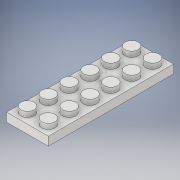
# Autodesk Inventor part: 2x6 short white pegged
Saved by Autodesk Inventor 2017 (Build 210142000, 142)
## iProperties
Created: 2018-05-09
Part Number: 2x6 short white pegged
Material: ABS Plastic
Document SubType Name: Modeling
Designer: Kyle
Density: 1.06 g/cm^3
Appearance: Smooth - White
Author: Kyle
Autodesk Inventor part; units mm, degrees
ref_plane "YZ Plane" through (0, 0, 0) normal (1, 0, 0) x (0, 1, 0)
ref_plane "XZ Plane" through (0, 0, 0) normal (0, 1, 0) x (-1, 0, 0)
ref_plane "XY Plane" through (0, 0, 0) normal (0, 0, 1) x (1, 0, 0)
sketch "Sketch1" plane through (0, 0, 0) normal (0, 1, 0) x (-1, 0, 0)
  line L0 (0, 0) -> (15.5956, 0)
  line L1 (15.5956, 0) -> (15.5956, -46.7868)
  line L2 (15.5956, -46.7868) -> (0, -46.7868)
  line L3 (0, -46.7868) -> (0, 0)
  dimension "d0" = 15.5956
  dimension "d7" = 46.7868
  constraints: 8 end point, 2 parallel, 1 horizontal, 1 perpendicular
  measures "d0" distance of L1.end L2.end
  measures "d7" distance of L0.end L1.end
extrude "Extrusion1" add sketch "Sketch1" along normal blind 3.236
sketch "Sketch2" plane through (0, 3.236, 0) normal (0, 1, 0) x (1, 0, 0)
  line L0 (-15.5956, 0) -> (0, 0) construction
  line L1 (-15.5956, 0) -> (-11.6967, 0) construction
  line L2 (-11.6967, 0) -> (-11.6967, 3.8989) construction
  line L3 (-11.6967, 3.8989) -> (-15.5956, 3.8989) construction
  line L4 (-15.5956, 3.8989) -> (-15.5956, 0) construction
  circle A0 centre (-11.6967, 3.8989) radius 2.4498
  dimension "d10" = 3.8989
  dimension "d11" = 3.8989
  dimension "d12" = 4.8997
  constraints: 8 end point, 2 parallel, 1 centre point, 1 coincident, 1 horizontal, 1 perpendicular
  measures "d10" distance of L3.end L2.end
  measures "d11" distance of L2.end L1.end
  measures "d12" diameter of A0
extrude "Extrusion2" add sketch "Sketch2" along normal blind 1.9837
pattern_linear "Rectangular Pattern1" count 6 spacing 7.7978 along (0, 0, -1) count 2 spacing 7.7978 along (1, 0, 0) of "Extrusion2"
shell "Shell1" thickness 1.4732 removed faces 1 at (-5.1985, 0, -31.1912)
sketch "Sketch3" plane through (-14.1224, 1.7628, -1.4732) normal (0, -1, 0) x (1, 0, 0)
  circle A0 centre (10.2235, -2.4257) radius 2.4498 construction
  circle A1 centre (2.4257, -10.2235) radius 2.4498 construction
  line L0 (10.2235, -2.4257) -> (2.4257, -10.2235) construction
  circle A2 centre (6.3246, -6.3246) radius 3.064
  circle A3 centre (6.3246, -6.3246) radius 2.4498
  point P0 (14.1224, 1.4732)
  dimension "d22" = 4.8997
  constraints: 2 centre point, 2 end point, 1 coincident, 1 midpoint
  measures "d22" diameter of A3
extrude "Extrusion3" add sketch "Sketch3" along normal up to surface (1.7628 mm away)
pattern_linear "Rectangular Pattern2" count 5 spacing 7.7978 along (0, 0, -1) of "Extrusion3"
equation "\"d0\" = 2 * d1"
equation "\"d7\" = 6 * d1"
equation "\"d8\" = d2"
equation "\"d10\" = 0.5 * d1"
equation "\"d11\" = 0.5 * d1"
equation "\"d12\" = d3"
equation "\"d13\" = d4"
equation "\"d17\" = d1"
equation "\"d20\" = d1"
equation "\"d21\" = d5"
equation "\"d22\" = d3"
equation "\"d23\" = d4"
equation "\"d27\" = d1"
equation "\"d1\" = 7.7978"
equation "\"d2\" = 3.23596"
equation "\"d3\" = 4.89966"
equation "\"d4\" = 1.98374"
equation "\"d5\" = 1.4732"
equation "\"d6\" = 1.23952"
body "Solid1"
